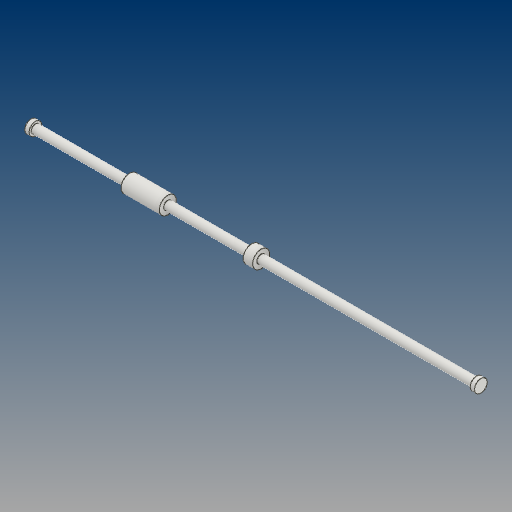
# Autodesk Inventor part: Shaft
Saved by Autodesk Inventor 2020 (Build 240168000, 168)
## iProperties
Created: 2020-08-26
Part Number: Shaft
Material: Steel
Document SubType Name: Modeling
Designer: alons
Density: 1 g/cm^3
Appearance: Steel
CustomPartVersion: 1
Author: alons
Length: 26.101 mm
Autodesk Inventor part; units mm, degrees
ref_plane "Start Plane" through (0, 0, 0) normal (1, 0, 0) x (0, 1, 0)
ref_plane "XZ Plane" through (0, 0, 0) normal (0, 1, 0) x (-1, 0, 0)
ref_plane "XY Plane" through (0, 0, 0) normal (0, 0, 1) x (1, 0, 0)
sketch "Main Sketch" plane through (0, 0, 0) normal (0, 0, 1) x (1, 0, 0)
  line L0 (0, 0) -> (26.101, 0)
  line L1 (0, 0) -> (0, 0.375)
  line L2 (0.25, 0.375) -> (0.25, 0.25)
  line L3 (0, 0.375) -> (0.25, 0.375)
  line L4 (5.715, 0.25) -> (5.715, 0.5)
  line L5 (0.25, 0.25) -> (5.715, 0.25)
  line L6 (7.932, 0.5) -> (7.932, 0.25)
  line L7 (5.715, 0.5) -> (7.932, 0.5)
  line L8 (7.932, 0.25) -> (12.804, 0.25)
  line L9 (13.351, 0.5) -> (13.351, 0.25)
  line L10 (12.804, 0.5) -> (13.351, 0.5)
  line L11 (13.351, 0.25) -> (25.851, 0.25)
  line L12 (25.851, 0.25) -> (25.851, 0.375)
  line L13 (26.101, 0.375) -> (26.101, 0)
  line L14 (25.851, 0.375) -> (26.101, 0.375)
  line L15 (12.804, 0.25) -> (12.804, 0.5)
  dimension "d3" = 0.75
  dimension "d6" = 0.5
  dimension "d7" = 1
  dimension "d8" = 0.5
  dimension "d9" = 1
  dimension "d10" = 0.5
  dimension "d11" = 0.75
  constraints: 32 end point, 8 vertical, 2 horizontal
  measures "d3" diameter of L3 L0
  measures "d6" diameter of L5 L0
  measures "d7" diameter of L7 L0
  measures "d8" diameter of L8 L0
  measures "d9" diameter of L10 L0
  measures "d10" diameter of L11 L0
  measures "d11" diameter of L14 L0
revolve "Revolution1" add sketch "Main Sketch" angle 360 about axis through (0, 0, 0) along (1, 0, 0)
fillet "Fillet1" [suppressed]
equation "\"Length\" = 26.101"
body "Solid1"
